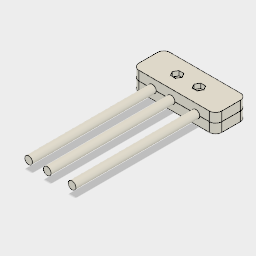
MoAgriS-Rod-Clamp v3 (Autodesk Fusion 360 design; units mm, degrees)
Autodesk Fusion 360 part; units mm, degrees
note: some values were not read from the file. Set by a fixed rule: which sketch regions a step uses.
sketch "Sketch1" plane through (0, 0, 0) normal (0, 0, 1) x (1, 0, 0)
  circle A0 centre (0, 0) radius 2.5
  circle A1 centre (12, 0) radius 2.5
  circle A2 centre (28, 0) radius 2.5
  dimension "d1" = 5
  dimension "d2" = 5
  dimension "d3" = 5
  dimension "d4" = 12
  dimension "d5" = 16
  measures "d1" diameter of A0
  measures "d2" diameter of A1
  measures "d3" diameter of A2
  measures "d4" distance of A0.centre A1.centre
  measures "d5" distance of A1.centre A2.centre
extrude "Extrude1" add sketch "Sketch1" along normal blind 100 makes body 1 at (2.4876, -0.2489, 33.3333) makes body 2 at (14.4876, -0.2489, 33.3333) makes body 3 at (30.4876, -0.2489, 33.3333)
sketch "Sketch2" plane through (0, 0, 0) normal (0, 1, 0) x (1, 0, 0)
  line L0 (-12.6637, -0.301) -> (40.7325, -0.301)
  line L1 (40.7325, -0.301) -> (40.7325, -20.301)
  line L2 (40.7325, -20.301) -> (-12.6637, -20.301)
  line L3 (-12.6637, -20.301) -> (-12.6637, -0.301)
  circle A0 centre (6, -10.301) radius 1.6
  circle A1 centre (20, -10.301) radius 1.6
  circle A2 centre (-8, -10.301) radius 1.6
  circle A3 centre (36, -10.301) radius 1.6
  dimension "d11" = 3.2
  dimension "d13" = 3.2
  dimension "d17" = 3.2
  dimension "d20" = 3.2
  dimension "d46" = 10
  dimension "d47" = 20
  measures "d11" diameter of A0
  measures "d13" diameter of A1
  measures "d17" diameter of A2
  measures "d20" diameter of A3
  measures "d46" distance of L0 A2.centre
  measures "d47" distance of L0 L2
extrude "Extrude2" add sketch "Sketch2" along normal blind 6 separate body contours L0 L1 L2 L3 | A0 | A1 | A2 | A3 makes body 4
combine "Combine1" operation cut target body 4 tool bodies 1 2 3 keep tools
extrude "Extrude3" cut sketch "Sketch2" along normal through all contours A0 | A1 bodies 4
mirror "Mirror1" about plane through (0, 0, 0) normal (0, -1, 0) of bodies 4 makes body 5
sketch "Sketch17" plane through (0, 6, 0) normal (0, 1, 0) x (-1, 0, 0)
  circle A0 centre (-20, 10.301) radius 1.6
  circle A1 centre (-6, 10.301) radius 1.6
  line L0 (12.6637, 20.301) -> (-40.7325, 20.301)
  line L1 (-40.7325, 20.301) -> (-40.7325, 0.301)
  line L2 (-40.7325, 0.301) -> (12.6637, 0.301)
  line L3 (12.6637, 0.301) -> (12.6637, 20.301)
  line L4 (-4.4203, 7.5463) -> (-2.8246, 10.2917)
  line L5 (-2.8246, 10.2917) -> (-4.4043, 13.0463)
  line L6 (-4.4043, 13.0463) -> (-7.5797, 13.0556)
  line L7 (-7.5797, 13.0556) -> (-9.1754, 10.3102)
  line L8 (-9.1754, 10.3102) -> (-7.5957, 7.5556)
  line L9 (-7.5957, 7.5556) -> (-4.4203, 7.5463)
  line L10 (-18.4065, 7.541) -> (-16.813, 10.301)
  line L11 (-16.813, 10.301) -> (-18.4065, 13.061)
  line L12 (-18.4065, 13.061) -> (-21.5935, 13.061)
  line L13 (-21.5935, 13.061) -> (-23.187, 10.301)
  line L14 (-23.187, 10.301) -> (-21.5935, 7.541)
  line L15 (-21.5935, 7.541) -> (-18.4065, 7.541)
  point P0 (-6, 10.301)
  point P1 (-20, 10.301)
  dimension "d134" = 2.75
  dimension "d135" = 2.76
  measures "d134" distance of P0 L9
  measures "d135" distance of P1 L15
chamfer "Chamfer3" distance 2 angle 45 2 edges at (4.5083, -6, 9.7224) (18.5083, -6, 9.7224) on bodies 5
extrude "Extrude11" cut sketch "Sketch17" against normal blind 3 contours A0 | A1 | L4 L5 L6 L7 L8 L9 | L10 L11 L12 L13 L14 L15 bodies 4
fillet "Fillet11" radius 4 8 edges at (-12.6637, 3, 0.301) (-12.6637, 3, 20.301) (40.7325, 3, 20.301) (40.7325, 3, 0.301) (-12.6637, -3, 0.301) (-12.6637, -3, 20.301) (40.7325, -3, 20.301) (40.7325, -3, 0.301) on bodies 4 5
equation "d11 = screws"
equation "d13 = screws"
equation "d17 = screws"
equation "d20 = screws"
equation "d46 = ( d47 / 2 )"
equation "screws = 3.2 mm"
equation "potHeight = 185 mm"
equation "potTopWidth = 205 mm"
equation "potBottomWidth = 135 mm"
equation "potShellWidth = 8.8 mm"
